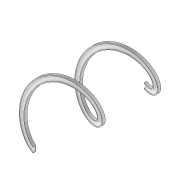
# Autodesk Inventor part: Spirale
Saved by Autodesk Inventor 2020 (Build 240168000, 168)
## iProperties
Created: 2020-04-19
Part Number: Spirale
Material: Generisch
Document SubType Name: Modeling
Designer: franz
Density: 1 g/cm^3
Appearance: Vorgabe
Author: franz
Autodesk Inventor part; units mm, degrees
ref_plane "YZ Plane" through (0, 0, 0) normal (1, 0, 0) x (0, 1, 0)
ref_plane "XZ Plane" through (0, 0, 0) normal (0, 1, 0) x (-1, 0, 0)
ref_plane "XY Plane" through (0, 0, 0) normal (0, 0, 1) x (1, 0, 0)
sketch "Skizze1" plane through (0, 0, 0) normal (1, 0, 0) x (0, 1, 0)
  arc A0 (-7.5, 0) -> (7.5, 0) centre (0, 0) ccw
  line L0 (7.5, 0) -> (10, 0)
  line L1 (10, 0) -> (10, -10)
  line L2 (10, -10) -> (-10, -10)
  line L3 (-10, -10) -> (-10, 0)
  line L4 (-10, 0) -> (-7.5, 0)
  line L5 (84.598, 14.8599) -> (84.598, -59.8609)
  line L6 (-28.9196, 0) -> (103.5177, 0) projected
  line L7 (0, -74.805) -> (0, 29.804) projected
  dimension "d8" = 7.5
  dimension "d9" = 20
  dimension "d10" = 10
  constraints: 12 end point, 3 vertical, 2 collinear, 2 point on circle, 1 centre point, 1 coincident, 1 parallel, 1 other
  measures "d8" radius of A0
  measures "d9" distance between parallel lines of L1 L3
  measures "d10" distance between parallel lines of L4 L2
coil "Spirale1" sketch "Skizze1" operation add axis through (0, 84.598, 14.8599) along (0, 0, -1) pitch 200 turns 2 hand right contours A0 L7 L2 L3 L4 | A0 L0 L1 L2 L7
